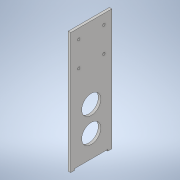
# Autodesk Inventor part: center_2Poke
Saved by Autodesk Inventor 2020 (Build 240168000, 168)
## iProperties
Created: 2018-12-12
Part Number: center_2Poke
Material: Generic
Document SubType Name: Modeling
Designer: aonih
Density: 1 g/cm^3
Appearance: Default
Author: aonih
Autodesk Inventor part; units mm, degrees
ref_plane "YZ Plane" through (0, 0, 0) normal (1, 0, 0) x (0, 1, 0)
ref_plane "XZ Plane" through (0, 0, 0) normal (0, 1, 0) x (-1, 0, 0)
ref_plane "XY Plane" through (0, 0, 0) normal (0, 0, 1) x (1, 0, 0)
sketch "Sketch1" plane through (0, 0, 0) normal (1, 0, 0) x (0, 1, 0)
  line L0 (128.3979, 81.9005) -> (-112.6021, 81.9005)
  line L1 (-112.6021, 81.9005) -> (-112.6021, -0.0995)
  line L2 (-112.6021, -0.0995) -> (128.3979, -0.0995)
  line L3 (128.3979, -0.0995) -> (128.3979, 81.9005)
  circle A0 centre (-45.6021, 40.9005) radius 19 construction
  line L4 (-112.6021, 73.9005) -> (-109.6021, 73.9005)
  line L5 (-109.6021, 73.9005) -> (-109.6021, 7.9005)
  line L6 (-109.6021, 7.9005) -> (-112.6021, 7.9005)
  line L7 (-112.6021, 7.9005) -> (-112.6021, 73.9005)
  circle A1 centre (111.4349, 69.7734) radius 2.5
  point P0 (0, 0)
  dimension "d0" = 241
  dimension "d1" = 82
  dimension "d2" = 38
  dimension "d3" = 41
  dimension "d4" = 174
  dimension "d5" = 66
  dimension "d6" = 3
  dimension "d7" = 8
  dimension "d24" = 5
  constraints: 16 end point, 4 parallel, 2 centre point, 2 horizontal, 2 perpendicular, 1 point on line
  measures "d0" distance of L1.end L2.end
  measures "d1" distance of L2.end L0.start
  measures "d2" diameter of A0
  measures "d3" distance from line of L0 A0.centre
  measures "d4" distance from line of L3 A0.centre
  measures "d5" distance of L4.end L5.end
  measures "d6" distance of L5.end L6.end
  measures "d7" distance from line of L2 L5.end
  measures "d24" diameter of A1
extrude "Extrusion3" add sketch "Sketch1" along normal blind 5 contours L3 L2 L1 L6 L5 L4 L0 | A1
sketch "Sketch3" plane through (5, 0, 0) normal (1, 0, 0) x (0, 0, -1)
  circle A0 centre (-65.9005, 108.8979) radius 2.5
  line L0 (-81.9005, 128.3979) -> (-81.9005, -112.6021) projected
  line L1 (-81.9005, 128.3979) -> (-74.525, 128.3979) construction
  line L2 (-81.9005, 122.7969) -> (-81.9005, 128.3979) construction
  circle A1 centre (-15.9005, 108.8979) radius 2.5
  circle A2 centre (-65.9005, 58.8979) radius 2.5
  circle A3 centre (-15.9005, 58.8979) radius 2.5
  line L3 (0.0995, -112.6021) -> (0.0995, 128.3979) projected
  line L4 (0.0995, 128.3979) -> (-81.9005, 128.3979) projected
  point P0 (0, 0)
  dimension "d25" = 5
  dimension "d28" = 50
  dimension "d31" = 50
  dimension "d34" = 82
  dimension "d35" = 16
  dimension "d36" = 19.5
  constraints: 4 centre point, 4 end point, 2 horizontal, 1 vertical, 6 other
  measures "d25" diameter of A0
  measures "d28" distance of A0.centre A1.centre
  measures "d31" distance of A0.centre A2.centre
  measures "d34" distance between parallel lines of L3 L0
  measures "d35" distance from line of L0 A2.centre
  measures "d36" distance from line of L4 A0.centre
extrude "Extrusion4" cut sketch "Sketch3" against normal up to surface (5 mm away)
sketch "Sketch4" plane through (5, 0, 0) normal (1, 0, 0) x (0, 0, -1)
  circle A0 centre (-40.9005, -65.6021) radius 19
  line L0 (-73.9005, -109.6021) -> (-7.9005, -109.6021) projected
  point P0 (0, 0)
  point P1 (-40.9005, -109.6021)
  dimension "d39" = 38
  dimension "d40" = 44
  constraints: 1 centre point, 1 midpoint, 1 vertical alignment
  measures "d39" diameter of A0
  measures "d40" distance from line of L0 A0.centre
extrude "Extrusion5" cut sketch "Sketch4" against normal up to surface (5 mm away)
pattern_linear "Rectangular Pattern1" count 2 spacing 50 along (0, 1, 0) of "Extrusion5"
equation "\"d3\" = 0.5 * d1"
equation "\"d7\" = -0.5 * d5 + 0.5 * d1"
equation "\"d35\" = -0.5 * d28 + 0.5 * d34"
body "Solid2"
